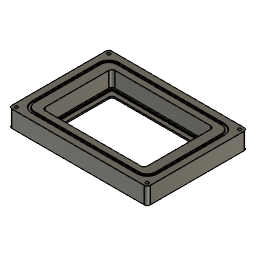
Base V3.0 (Autodesk Fusion 360 design; units mm, degrees)
part number: 2026-01-30-14-30-51-369
Autodesk Fusion 360 part; units mm, degrees
note: some values were not read from the file. Set by a fixed rule: which sketch regions a step uses.
sketch "Sketch1" plane through (0, 0, 0) normal (0, 0, 1) x (1, 0, 0)
  line L0 (86, -65) -> (-86, -65)
  line L1 (-90, -61) -> (-90, 61)
  line L2 (-86, 65) -> (86, 65)
  line L3 (90, 61) -> (90, -61)
  line L4 (90, -65) -> (-90, 65) construction
  line L5 (-90, -65) -> (90, 65) construction
  arc A0 (-86, 65) -> (-90, 61) centre (-86, 61) ccw
  arc A1 (90, 61) -> (86, 65) centre (86, 61) ccw
  arc A2 (86, -65) -> (90, -61) centre (86, -61) ccw
  arc A3 (-90, -61) -> (-86, -65) centre (-86, -61) ccw
  circle A4 centre (-85, 60) radius 2
  line L6 (0, 65) -> (0, -65) construction
  line L7 (90, 0) -> (-90, 0) construction
  circle A5 centre (85, 60) radius 2
  circle A6 centre (85, -60) radius 2
  circle A7 centre (-85, -60) radius 2
  dimension "d1" = 180
  dimension "d2" = 130
  dimension "d26" = 4
  dimension "d27" = 4
  dimension "d28" = 4
  dimension "d29" = 4
  dimension "d30" = 4
  dimension "d31" = 5
  dimension "d32" = 5
  constraint horizontal L0
  constraint perpendicular L0 L1
  constraint parallel L0 L2
  constraint parallel L1 L3
  constraint coincident L4 origin
  constraint coincident L5 origin
  constraint coincident L4.end L2
  constraint coincident L4.end L1
  constraint tangent L2 A0
  constraint tangent L1 A0
  constraint coincident L5.end L3
  constraint coincident L5.end L2
  constraint tangent L3 A1
  constraint tangent L2 A1
  constraint coincident L4.start L3
  constraint coincident L4.start L0
  constraint tangent L3 A2
  constraint tangent L0 A2
  constraint coincident L5.start L1
  constraint coincident L5.start L0
  constraint tangent L1 A3
  constraint tangent L0 A3
  constraint midpoint L2 L6.start
  constraint midpoint L0 L6.end
  constraint midpoint L3 L7.start
  constraint midpoint L1 L7.end
  constraint symmetric A4 L6 A5
  constraint symmetric A4 L7 A7
  constraint symmetric L7 A5 A6
  measures "d1" distance of L4.end L5.end
  measures "d2" distance of L5.start L4.end
  measures "d26" radius of A0
  measures "d27" radius of A1
  measures "d28" radius of A2
  measures "d29" radius of A3
  measures "d30" diameter of A4
  measures "d31" distance of L2 A4.centre
  measures "d32" distance of L1 A4.centre
extrude "Extrude1" add sketch "Sketch1" along normal blind 22
sketch "Sketch2" plane through (0, 0, 22) normal (0, 0, 1) x (-1, 0, 0)
  line L0 (-86, -65) -> (86, -65)
  line L1 (90, -61) -> (90, 61)
  line L2 (86, 65) -> (-86, 65)
  line L3 (-90, 61) -> (-90, -61)
  line L4 (-62.2, 45.25) -> (62.2, 45.25)
  line L5 (66.2, 41.25) -> (66.2, -41.25)
  line L6 (62.2, -45.25) -> (-62.2, -45.25)
  line L7 (-66.2, -41.25) -> (-66.2, 41.25)
  line L8 (-66.2, 45.25) -> (66.2, -45.25) construction
  line L9 (66.2, 45.25) -> (-66.2, -45.25) construction
  arc A0 (86, -65) -> (90, -61) centre (86, -61) ccw
  arc A1 (90, 61) -> (86, 65) centre (86, 61) ccw
  arc A2 (-86, 65) -> (-90, 61) centre (-86, 61) ccw
  arc A3 (-90, -61) -> (-86, -65) centre (-86, -61) ccw
  circle A4 centre (85, 60) radius 2
  circle A5 centre (-85, 60) radius 2
  circle A6 centre (-85, -60) radius 2
  circle A7 centre (85, -60) radius 2
  arc A8 (62.2, -45.25) -> (66.2, -41.25) centre (62.2, -41.25) ccw
  arc A9 (-66.2, -41.25) -> (-62.2, -45.25) centre (-62.2, -41.25) ccw
  arc A10 (66.2, 41.25) -> (62.2, 45.25) centre (62.2, 41.25) ccw
  arc A11 (-62.2, 45.25) -> (-66.2, 41.25) centre (-62.2, 41.25) ccw
  dimension "d5" = 132.4
  dimension "d6" = 90.5
  dimension "d52" = 4
  dimension "d53" = 4
  dimension "d54" = 4
  dimension "d55" = 4
  constraint horizontal L4
  constraint perpendicular L4 L5
  constraint parallel L4 L6
  constraint parallel L5 L7
  constraint coincident L8 origin
  constraint coincident L9 origin
  constraint coincident L8.end L6
  constraint coincident L8.end L5
  constraint tangent L6 A8
  constraint tangent L5 A8
  constraint coincident L9.end L6
  constraint coincident L9.end L7
  constraint tangent L6 A9
  constraint tangent L7 A9
  constraint coincident L9.start L5
  constraint coincident L9.start L4
  constraint tangent L5 A10
  constraint tangent L4 A10
  constraint coincident L8.start L7
  constraint coincident L8.start L4
  constraint tangent L7 A11
  constraint tangent L4 A11
  measures "d5" distance of L8.end L9.end
  measures "d6" distance of L9.start L8.end
  measures "d52" radius of A8
  measures "d53" radius of A9
  measures "d54" radius of A10
  measures "d55" radius of A11
extrude "Extrude2" cut sketch "Sketch2" against normal blind 20 contours L4 L5 L6 L7 A8 A9 A10 A11
sketch "Sketch3" plane through (0, 0, 22) normal (0, 0, 1) x (-1, 0, 0)
  line L0 (66.2, 41.25) -> (66.2, -41.25)
  line L1 (62.2, -45.25) -> (-62.2, -45.25)
  line L2 (-66.2, -41.25) -> (-66.2, 41.25)
  line L3 (-62.2, 45.25) -> (62.2, 45.25)
  line L4 (-86, -65) -> (86, -65)
  line L5 (90, -61) -> (90, 61)
  line L6 (86, 65) -> (-86, 65)
  line L7 (-90, 61) -> (-90, -61)
  line L8 (-79.9494, 54.9494) -> (79.9494, 54.9494) construction
  line L9 (79.9494, 54.9494) -> (79.9494, -54.9494) construction
  line L10 (79.9494, -54.9494) -> (-79.9494, -54.9494) construction
  line L11 (-79.9494, -54.9494) -> (-79.9494, 54.9494) construction
  line L12 (-79.9494, 54.9494) -> (79.9494, -54.9494) construction
  line L13 (79.9494, 54.9494) -> (-79.9494, -54.9494) construction
  line L14 (78.5149, 43.2459) -> (78.5149, -43.2459)
  line L15 (68.2459, -53.5149) -> (-68.2459, -53.5149)
  line L16 (-78.5149, -43.2459) -> (-78.5149, 43.2459)
  line L17 (-69.5341, 47.3937) -> (78.5149, -53.5149) construction
  line L18 (70.6619, 45.6619) -> (-70.6619, -45.6619) construction
  line L19 (-68.2459, 56.3839) -> (68.2459, 56.3839)
  line L20 (81.3839, 43.2459) -> (81.3839, -43.2459)
  line L21 (68.2459, -56.3839) -> (-68.2459, -56.3839)
  line L22 (-81.3839, -43.2459) -> (-81.3839, 43.2459)
  line L23 (-72.429, 50.1798) -> (81.3839, -56.3839) construction
  line L24 (73.5309, 48.5309) -> (-73.5309, -48.5309) construction
  arc A0 (68.2459, -53.5149) -> (78.5149, -43.2459) centre (68.2459, -43.2459) ccw
  arc A1 (68.2459, -56.3839) -> (81.3839, -43.2459) centre (68.2459, -43.2459) ccw
  line L25 (0, -65) -> (0, 65) construction
  line L26 (-90, 0) -> (90, 0) construction
  arc A2 (-78.5149, -43.2459) -> (-68.2459, -53.5149) centre (-68.2459, -43.2459) ccw
  arc A3 (-81.3839, -43.2459) -> (-68.2459, -56.3839) centre (-68.2459, -43.2459) ccw
  arc A4 (-68.2459, 53.5149) -> (-78.5149, 43.2459) centre (-68.2459, 43.2459) ccw
  arc A5 (-68.2459, 56.3839) -> (-81.3839, 43.2459) centre (-68.2459, 43.2459) ccw
  arc A6 (78.5149, 43.2459) -> (68.2459, 53.5149) centre (68.2459, 43.2459) ccw
  arc A7 (81.3839, 43.2459) -> (68.2459, 56.3839) centre (68.2459, 43.2459) ccw
  line L27 (-68.2459, 53.5149) -> (68.2459, 53.5149)
  arc A8 (86, -65) -> (90, -61) centre (86, -61) ccw
  arc A9 (90, 61) -> (86, 65) centre (86, 61) ccw
  arc A10 (-86, 65) -> (-90, 61) centre (-86, 61) ccw
  arc A11 (-90, -61) -> (-86, -65) centre (-86, -61) ccw
  circle A12 centre (85, 60) radius 2
  circle A13 centre (-85, 60) radius 2
  circle A14 centre (-85, -60) radius 2
  circle A15 centre (85, -60) radius 2
  arc A16 (66.2, 41.25) -> (62.2, 45.25) centre (62.2, 41.25) ccw
  arc A17 (62.2, -45.25) -> (66.2, -41.25) centre (62.2, -41.25) ccw
  arc A18 (-66.2, -41.25) -> (-62.2, -45.25) centre (-62.2, -41.25) ccw
  arc A19 (-62.2, 45.25) -> (-66.2, 41.25) centre (-62.2, 41.25) ccw
  dimension "d9" = 159.8988
  dimension "d15" = 109.8988
  dimension "d16" = 1.4345
  dimension "d17" = 1.4345
  dimension "d18" = 1.4345
  dimension "d19" = 1.4345
  dimension "d20" = 10.269
  dimension "d21" = 13.138
  constraint horizontal L8
  constraint perpendicular L8 L9
  constraint parallel L8 L10
  constraint parallel L9 L11
  constraint coincident L12 origin
  constraint coincident L13 origin
  constraint parallel L15 L27
  constraint parallel L14 L16
  constraint coincident L17 origin
  constraint coincident L18 origin
  constraint horizontal L19
  constraint perpendicular L19 L20
  constraint parallel L19 L21
  constraint parallel L20 L22
  constraint coincident L23 origin
  constraint coincident L24 origin
  constraint coincident L17.end L15
  constraint coincident L17.end L14
  constraint tangent L15 A0
  constraint tangent L14 A0
  constraint coincident L23.end L21
  constraint coincident L23.end L20
  constraint tangent L21 A1
  constraint tangent L20 A1
  constraint midpoint L4 L25.start
  constraint midpoint L6 L25.end
  constraint midpoint L7 L26.start
  constraint midpoint L5 L26.end
  constraint symmetric L15.start L25 L15.end
  constraint symmetric L14.end L25 L16.start
  constraint symmetric A0 L25 A2
  constraint symmetric L21.start L25 L21.end
  constraint symmetric L20.end L25 L22.start
  constraint symmetric A1 L25 A3
  constraint symmetric L15.start L26 A6.end
  constraint symmetric L14.end L26 L14.start
  constraint symmetric A0 L26 A6
  constraint symmetric L21.start L26 L19.end
  constraint symmetric L20.end L26 L20.start
  constraint symmetric A1 L26 A7
  constraint symmetric L26 L15.end A4.start
  constraint symmetric L26 L16.start L16.end
  constraint symmetric L26 A2 A4
  constraint symmetric L26 L21.end L19.start
  constraint symmetric L26 L22.start L22.end
  constraint symmetric L26 A3 A5
  measures "d9" distance of L8.start L8.end
  measures "d15" distance of L8 L10
  measures "d16" distance of L11 L16
  measures "d17" distance of L10 L15
  measures "d18" distance of L11 L22
  measures "d19" distance of L10 L21
  measures "d20" radius of A0
  measures "d21" radius of A1
extrude "Extrude3" cut sketch "Sketch3" against normal blind 1.424 contours L19 L20 L21 L22 A1 A3 A5 A7
draft "Draft1" angle 10 neutral plane through (0, 0, 20.576) pull (0, 0, 1) 16 faces at (-78.5149, -14.4153, 21.5253) (-70.6669, 53.2254, 21.0507) (-22.7486, 53.5149, 21.5253) (74.2025, 51.6108, 21.0507) (78.5149, 14.4153, 21.0507) (71.6046, -52.9501, 21.5253) (22.7486, -53.5149, 21.5253) (-70.6669, -53.2254, 21.0507) (-81.3839, -14.4153, 21.5253) (-68.871, -56.369, 21.0507) (22.7486, -56.3839, 21.0507) (77.7543, -52.3122, 21.0507) (81.3839, 14.4153, 21.5253) (77.3122, 52.7543, 21.0507) (-22.7486, 56.3839, 21.0507) (-73.1288, 55.4428, 21.0507)
sketch "Sketch4" plane through (0, 0, 2) normal (0, 0, 1) x (-1, 0, 0)
  line L0 (-62.2, -45.25) -> (62.2, -45.25)
  line L1 (66.2, -41.25) -> (66.2, 41.25)
  line L2 (62.2, 45.25) -> (-62.2, 45.25)
  line L3 (-66.2, 41.25) -> (-66.2, -41.25)
  line L4 (-52.2, 35.25) -> (52.2, 35.25)
  line L5 (56.2, 31.25) -> (56.2, -31.25)
  line L6 (52.2, -35.25) -> (-52.2, -35.25)
  line L7 (-56.2, -31.25) -> (-56.2, 31.25)
  line L8 (-56.2, 35.25) -> (56.2, -35.25) construction
  line L9 (56.2, 35.25) -> (-56.2, -35.25) construction
  arc A0 (66.2, 41.25) -> (62.2, 45.25) centre (62.2, 41.25) ccw
  arc A1 (-62.2, 45.25) -> (-66.2, 41.25) centre (-62.2, 41.25) ccw
  arc A2 (-66.2, -41.25) -> (-62.2, -45.25) centre (-62.2, -41.25) ccw
  arc A3 (62.2, -45.25) -> (66.2, -41.25) centre (62.2, -41.25) ccw
  arc A4 (52.2, -35.25) -> (56.2, -31.25) centre (52.2, -31.25) ccw
  arc A5 (-56.2, -31.25) -> (-52.2, -35.25) centre (-52.2, -31.25) ccw
  arc A6 (-52.2, 35.25) -> (-56.2, 31.25) centre (-52.2, 31.25) ccw
  arc A7 (56.2, 31.25) -> (52.2, 35.25) centre (52.2, 31.25) ccw
  dimension "d35" = 10
  dimension "d36" = 10
  dimension "d71" = 4
  dimension "d72" = 4
  dimension "d73" = 4
  dimension "d74" = 4
  constraint horizontal L4
  constraint perpendicular L4 L5
  constraint parallel L4 L6
  constraint parallel L5 L7
  constraint coincident L8 origin
  constraint coincident L9 origin
  constraint coincident L8.end L6
  constraint coincident L8.end L5
  constraint tangent L6 A4
  constraint tangent L5 A4
  constraint coincident L9.end L6
  constraint coincident L9.end L7
  constraint tangent L6 A5
  constraint tangent L7 A5
  constraint coincident L8.start L7
  constraint coincident L8.start L4
  constraint tangent L7 A6
  constraint tangent L4 A6
  constraint coincident L9.start L4
  constraint coincident L9.start L5
  constraint tangent L4 A7
  constraint tangent L5 A7
  measures "d35" distance of L3 L7
  measures "d36" distance of L0 L6
  measures "d71" radius of A4
  measures "d72" radius of A5
  measures "d73" radius of A6
  measures "d74" radius of A7
extrude "Extrude4" cut sketch "Sketch4" against normal blind 5 contours L4 L5 L6 L7 A4 A5 A6 A7
sketch "Sketch6" plane through (0, 0, 2) normal (0, 0, 1) x (-1, 0, 0)
  line L0 (56.2, 31.25) -> (56.2, -31.25)
  line L1 (52.2, -35.25) -> (-52.2, -35.25)
  line L2 (-56.2, -31.25) -> (-56.2, 31.25)
  line L3 (-52.2, 35.25) -> (52.2, 35.25)
  arc A0 (66.2, 41.25) -> (62.2, 45.25) centre (62.2, 41.25) ccw
  line L4 (62.2, 45.25) -> (-62.2, 45.25)
  arc A1 (-62.2, 45.25) -> (-66.2, 41.25) centre (-62.2, 41.25) ccw
  line L5 (-66.2, 41.25) -> (-66.2, -41.25)
  arc A2 (-66.2, -41.25) -> (-62.2, -45.25) centre (-62.2, -41.25) ccw
  line L6 (-62.2, -45.25) -> (62.2, -45.25)
  arc A3 (62.2, -45.25) -> (66.2, -41.25) centre (62.2, -41.25) ccw
  line L7 (66.2, -41.25) -> (66.2, 41.25)
  arc A4 (60.9079, -41.3399) -> (62.4799, -39.7679) centre (60.9079, -39.7679) ccw construction
  arc A5 (-62.4799, -39.7399) -> (-60.9079, -41.3119) centre (-60.9079, -39.7399) ccw construction
  line L8 (-48.9575, -41.8399) -> (48.9575, -41.8399) construction
  line L9 (48.9575, 41.8399) -> (-48.9575, 41.8399) construction
  line L10 (-62.9799, 29.7119) -> (-62.9799, 27.8175) construction
  line L11 (48.9575, -41.8399) -> (50.8519, -41.8399) construction
  line L12 (62.4799, 30.3078) -> (62.4799, 39.7679) construction
  arc A6 (-60.88, 42.74) -> (-63.88, 39.74) centre (-60.88, 39.74) ccw construction
  line L13 (63.88, 39.74) -> (63.88, -39.74) construction
  arc A7 (63.88, 39.74) -> (60.88, 42.74) centre (60.88, 39.74) ccw construction
  line L14 (-62.9799, -29.7119) -> (-62.4799, -30.3078) construction
  line L15 (51.4478, 41.3399) -> (50.8519, 41.8399) construction
  arc A8 (60.88, -42.74) -> (63.88, -39.74) centre (60.88, -39.74) ccw construction
  line L16 (-48.9575, 41.8399) -> (-50.8519, 41.8399) construction
  line L17 (-60.88, 42.74) -> (60.88, 42.74) construction
  line L18 (-62.9799, -27.8175) -> (-62.9799, -29.7119) construction
  line L19 (60.88, -42.74) -> (-60.88, -42.74) construction
  line L20 (62.9799, 29.7119) -> (62.4799, 30.3078) construction
  line L21 (-50.8519, 41.8399) -> (-51.4811, 41.3119) construction
  line L22 (62.4799, -39.7679) -> (62.4799, -30.3078) construction
  line L23 (-50.8519, -41.8399) -> (-48.9575, -41.8399) construction
  line L24 (60.9079, 41.3399) -> (51.4478, 41.3399) construction
  line L25 (50.8519, 41.8399) -> (48.9575, 41.8399) construction
  line L26 (62.9799, 27.8175) -> (62.9799, 29.7119) construction
  line L27 (51.4478, -41.3399) -> (60.9079, -41.3399) construction
  line L28 (62.9799, -27.8175) -> (62.9799, 27.8175) construction
  line L29 (-63.88, -39.74) -> (-63.88, 39.74) construction
  line L30 (50.8519, -41.8399) -> (51.4478, -41.3399) construction
  line L31 (62.9799, -29.7119) -> (62.9799, -27.8175) construction
  arc A9 (-63.88, -39.74) -> (-60.88, -42.74) centre (-60.88, -39.74) ccw construction
  arc A10 (62.4799, 39.7679) -> (60.9079, 41.3399) centre (60.9079, 39.7679) ccw construction
  line L32 (62.4799, -30.3078) -> (62.9799, -29.7119) construction
  line L33 (-62.4799, 30.3078) -> (-62.9799, 29.7119) construction
  line L34 (-60.9079, -41.3119) -> (-51.4811, -41.3119) construction
  arc A11 (-60.9079, 41.3119) -> (-62.4799, 39.7399) centre (-60.9079, 39.7399) ccw construction
  line L35 (-51.4811, -41.3119) -> (-50.8519, -41.8399) construction
  line L36 (-51.4811, 41.3119) -> (-60.9079, 41.3119) construction
  line L37 (-62.4799, 39.7399) -> (-62.4799, 30.3078) construction
  line L38 (-62.4799, -30.3078) -> (-62.4799, -39.7399) construction
  line L39 (-62.9799, 27.8175) -> (-62.9799, -27.8175) construction
  line L40 (0, -45.25) -> (0, 45.25) construction
  line L41 (-66.2, 0) -> (66.2, 0) construction
  line L42 (-60.85, 43.25) -> (60.85, 43.25)
  line L43 (64.35, 39.75) -> (64.35, -39.75)
  line L44 (60.85, -43.25) -> (-60.85, -43.25)
  line L45 (-64.35, -39.75) -> (-64.35, 39.75)
  line L46 (-64.35, 43.25) -> (64.35, -43.25) construction
  line L47 (64.35, 43.25) -> (-64.35, -43.25) construction
  arc A12 (60.85, -43.25) -> (64.35, -39.75) centre (60.85, -39.75) ccw
  arc A13 (-64.35, -39.75) -> (-60.85, -43.25) centre (-60.85, -39.75) ccw
  arc A14 (-60.85, 43.25) -> (-64.35, 39.75) centre (-60.85, 39.75) ccw
  arc A15 (64.35, 39.75) -> (60.85, 43.25) centre (60.85, 39.75) ccw
  line L48 (-60.85, 40.75) -> (60.85, 40.75)
  line L49 (61.85, 39.75) -> (61.85, -39.75)
  line L50 (60.85, -40.75) -> (-60.85, -40.75)
  line L51 (-61.85, -39.75) -> (-61.85, 39.75)
  line L52 (-61.85, 40.75) -> (61.85, -40.75) construction
  line L53 (61.85, 40.75) -> (-61.85, -40.75) construction
  arc A16 (-61.85, -39.75) -> (-60.85, -40.75) centre (-60.85, -39.75) ccw
  arc A17 (60.85, -40.75) -> (61.85, -39.75) centre (60.85, -39.75) ccw
  arc A18 (61.85, 39.75) -> (60.85, 40.75) centre (60.85, 39.75) ccw
  arc A19 (-60.85, 40.75) -> (-61.85, 39.75) centre (-60.85, 39.75) ccw
  arc A20 (52.2, -35.25) -> (56.2, -31.25) centre (52.2, -31.25) ccw
  arc A21 (-56.2, -31.25) -> (-52.2, -35.25) centre (-52.2, -31.25) ccw
  arc A22 (-52.2, 35.25) -> (-56.2, 31.25) centre (-52.2, 31.25) ccw
  arc A23 (56.2, 31.25) -> (52.2, 35.25) centre (52.2, 31.25) ccw
  dimension "d56" = 128.7
  dimension "d57" = 86.5
  dimension "d58" = 3.5
  dimension "d59" = 3.5
  dimension "d60" = 3.5
  dimension "d61" = 3.5
  dimension "d63" = 2.5
  dimension "d64" = 2.5
  dimension "d65" = 1
  dimension "d66" = 1
  dimension "d67" = 1
  dimension "d68" = 1
  constraint midpoint L6 L40.start
  constraint midpoint L4 L40.end
  constraint midpoint L5 L41.start
  constraint midpoint L7 L41.end
  constraint horizontal L42
  constraint perpendicular L42 L43
  constraint parallel L42 L44
  constraint parallel L43 L45
  constraint coincident L46 origin
  constraint coincident L47 origin
  constraint coincident L46.end L44
  constraint coincident L46.end L43
  constraint tangent L44 A12
  constraint tangent L43 A12
  constraint coincident L47.end L45
  constraint coincident L47.end L44
  constraint tangent L45 A13
  constraint tangent L44 A13
  constraint coincident L46.start L45
  constraint coincident L46.start L42
  constraint tangent L45 A14
  constraint tangent L42 A14
  constraint coincident L47.start L42
  constraint coincident L47.start L43
  constraint tangent L42 A15
  constraint tangent L43 A15
  constraint horizontal L48
  constraint perpendicular L48 L49
  constraint parallel L48 L50
  constraint parallel L49 L51
  constraint coincident L52 origin
  constraint coincident L53 origin
  constraint coincident L53.end L51
  constraint coincident L53.end L50
  constraint tangent L51 A16
  constraint tangent L50 A16
  constraint coincident L52.end L50
  constraint coincident L52.end L49
  constraint tangent L50 A17
  constraint tangent L49 A17
  constraint coincident L53.start L48
  constraint coincident L53.start L49
  constraint tangent L48 A18
  constraint tangent L49 A18
  constraint coincident L52.start L51
  constraint coincident L52.start L48
  constraint tangent L51 A19
  constraint tangent L48 A19
  measures "d56" distance of L46.end L47.end
  measures "d57" distance of L47.start L46.end
  measures "d58" radius of A12
  measures "d59" radius of A13
  measures "d60" radius of A14
  measures "d61" radius of A15
  measures "d63" distance of L45 L51
  measures "d64" distance of L44 L50
  measures "d65" radius of A16
  measures "d66" radius of A17
  measures "d67" radius of A18
  measures "d68" radius of A19
extrude "Extrude6" cut sketch "Sketch6" against normal blind 1 contours L42 L43 L44 L45 A12 A13 A14 A15
equation "d9 = ( ORingPerimeter - 100 mm ) / 4 + 50 mm"
equation "ORingDiameter = 1.78 mm" comment "Diamter of the O ring"
equation "ORingInnerDiameter = 170 mm" comment "Inner diamter of the o ring bore"
equation "ORingPerimeter = 2 * 3.1412 * ( ( ORingInnerDiameter / 2 ) + ORingDiameter / 2 )"
equation "PanelWidth = 80 mm"
equation "PanelLength = 115 mm"
equation "d15 = ( ORingPerimeter - 100 mm ) / 4"
equation "d16 = ( ( ORingDiameter * 1.05 ) / 2 ) + 0.5 mm"
equation "d17 = ( ( ORingDiameter * 1.05 ) / 2 ) + 0.5 mm"
equation "d18 = ( ( ORingDiameter * 1.05 ) / 2 ) + 0.5 mm"
equation "d19 = ( ( ORingDiameter * 1.05 ) / 2 ) + 0.5 mm"
equation "d20 = ( ORingDiameter ) * 6 + ORingDiameter * 0.05 - 0.5 mm"
equation "d21 = ( ORingDiameter ) * 6 + ( ORingDiameter * 1.1 ) + 0.5 mm"
equation "d22 = -ORingDiameter * 0.8"
equation "ORing2Diameter = 2 mm" comment "Second O ring Diameter"
equation "ORing2InnerDiameter = 126 mm" comment "Inner diameter of the second O Ring"
equation "ORing2Perimeter = 2 * 3.1412 * ( ( ORing2InnerDiameter / 2 ) + ORing2Diameter / 2 )"
